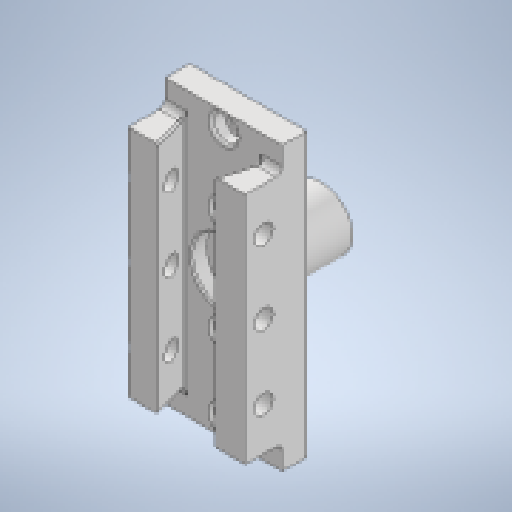
# Autodesk Inventor part: finger_adaptor
Saved by Autodesk Inventor 2024.3 (Build 283343010, 343A)
## iProperties
Created: 2025-06-26
Part Number: finger_adaptor
Material: 一般
Document SubType Name: Modeling
Designer: kshau
Density: 1 g/cm^3
Appearance: 滑らか - 黒
Author: kshau
Autodesk Inventor part; units mm, degrees
ref_plane "YZ Plane" through (0, 0, 0) normal (1, 0, 0) x (0, 1, 0)
ref_plane "XZ Plane" through (0, 0, 0) normal (0, 1, 0) x (-1, 0, 0)
ref_plane "XY Plane" through (0, 0, 0) normal (0, 0, 1) x (1, 0, 0)
sketch "スケッチ1" plane through (0, 0, 0) normal (0, 1, 0) x (-1, 0, 0)
  line L0 (0, 0) -> (19.05, 0)
  line L1 (19.05, 0) -> (19.05, 10)
  line L2 (19.05, 10) -> (0, 10)
  line L3 (0, 10) -> (0, 0)
  line L4 (19.05, 4) -> (0, 4)
  line L5 (14.265, 10) -> (15.873, 4)
  line L6 (9.525, 10) -> (9.525, 4)
  line L7 (0, 4) -> (19.05, 4)
  line L8 (4.785, 10) -> (3.177, 4)
  point P0 (3.177, 4)
  point P1 (4.785, 10)
  dimension "d0" = 19.05
  dimension "d1" = 10
  dimension "d2" = 4.785
  dimension "d3" = 4
  dimension "d4" = 3.177
  constraints: 18 end point, 5 point on line, 4 symmetric about line, 2 midpoint, 2 parallel, 2 perpendicular, 1 horizontal
  measures "d0" distance of L0.start L0.end
  measures "d1" distance of L0.end L1.end
  measures "d2" distance from line of L1 L5.start
  measures "d3" distance between parallel lines of L4 L0
  measures "d4" distance from line of L1 L5.end
extrude "押し出し1" add sketch "スケッチ1" along normal blind 46 contours L3 L4 L1 L0 | L3 L2 L8 L4 | L4 L5 L2 L1
sketch "スケッチ2" plane through (0, 0, 0) normal (0, 0, -1) x (-1, 0, 0)
  line L0 (15.873, 46) -> (3.177, 46) projected
  line L1 (9.525, 46) -> (9.525, 0)
  line L2 (15.873, 0) -> (3.177, 0) projected
  circle A0 centre (9.525, 23) radius 5
  point P0 (0, 0)
  dimension "d7" = 10
  constraints: 3 midpoint, 2 end point, 1 centre point
  measures "d7" diameter of A0
extrude "押し出し2" add sketch "スケッチ2" along normal blind 12.5
sketch "スケッチ3" plane through (-9.525, 23, -12.5) normal (0, 0, -1) x (-1, 0, 0)
  circle A0 centre (0, 0) radius 5 projected
  point P0 (-9.525, -23)
  constraints: 1 coincident
hole "穴1" at (-9.525, 23, -12.5) direction (0, 0, 1) diameter 3.1 end through all
sketch "スケッチ4" plane through (0, 0, 0) normal (0, 0, -1) x (-1, 0, 0)
  line L0 (15.873, 46) -> (3.177, 46) projected
  line L1 (9.525, 46) -> (9.525, 0)
  line L2 (15.873, 0) -> (3.177, 0) projected
  line L3 (0, 0) -> (0, 46) projected
  line L4 (0, 23) -> (19.05, 23)
  line L5 (19.05, 0) -> (19.05, 46) projected
  point P0 (9.525, 43.5)
  point P1 (9.525, 31.5)
  point P2 (9.525, 2.5)
  point P3 (9.525, 14.5)
  dimension "d17" = 2.5
  dimension "d18" = 12
  constraints: 4 end point, 4 midpoint, 2 point on line, 2 symmetric about line
  measures "d17" distance from line of L0 point (9.525, 43.5)
  measures "d18" distance of point (9.525, 43.5) point (9.525, 31.5)
hole "穴2" at (-9.525, 43.5, 0) at (-9.525, 31.5, 0) at (-9.525, 2.5, 0) at (-9.525, 14.5, 0) direction (0, 0, 1) diameter 2.1 end through all
sketch "スケッチ5" plane through (-19.05, 0, 0) normal (-1, 0, 0) x (0, 0, 1)
  line L0 (0, 46) -> (10, 46) projected
  line L1 (7, 46) -> (7, 0)
  line L2 (10, 0) -> (10, 46) projected
  line L3 (0, 0) -> (10, 0) projected
  line L4 (7, 23) -> (10, 23)
  point P0 (7, 11)
  point P1 (7, 35)
  dimension "d26" = 3
  dimension "d29" = 12
  constraints: 4 end point, 2 midpoint, 2 point on line, 1 coincident, 1 perpendicular, 1 symmetric about line, 1 vertical
  measures "d26" distance between parallel lines of L2 L1
  measures "d29" distance from line of point (7, 11) L4
hole "穴3" at (-19.05, 11, 7) at (-19.05, 23, 7) at (-19.05, 35, 7) direction (1, 0, 0) diameter 3.1 end through all countersink diameter 6.3 countersink angle 90
sketch "スケッチ6" plane through (-15.873, 0, 4) normal (0, 0, 1) x (1, 0, 0)
  circle A0 centre (6.348, 43.5) radius 1.05 projected
  circle A1 centre (6.348, 43.5) radius 2
  circle A2 centre (6.348, 31.5) radius 1.05 projected
  circle A3 centre (6.348, 31.5) radius 2
  circle A4 centre (6.348, 23) radius 1.55 projected
  circle A5 centre (6.348, 23) radius 3
  circle A6 centre (6.348, 14.5) radius 1.05 projected
  circle A7 centre (6.348, 14.5) radius 2
  circle A8 centre (6.348, 2.5) radius 1.05 projected
  circle A9 centre (6.348, 2.5) radius 2
  point P0 (15.873, 0)
  dimension "d37" = 4
  dimension "d38" = 4
  dimension "d39" = 6
  dimension "d40" = 4
  dimension "d41" = 4
  constraints: 5 centre point, 5 coincident
  measures "d37" diameter of A1
  measures "d38" diameter of A3
  measures "d39" diameter of A5
  measures "d40" diameter of A7
  measures "d41" diameter of A9
extrude "押し出し3" cut sketch "スケッチ6" against normal blind 2.1 contours A0 | A1 | A2 | A3 | A7 | A9
sketch "スケッチ7" plane through (0, 46, 0) normal (0, 1, 0) x (1, 0, 0)
  line L0 (-19.05, -10) -> (-14.265, -10) projected
  line L1 (-19.05, -10) -> (0, -10)
  line L2 (0, -10) -> (0, 0)
  line L3 (0, 0) -> (-19.05, 0)
  line L4 (-19.05, 0) -> (-19.05, -10)
  line L5 (-19.05, -4) -> (0, -4)
  line L6 (0, -10) -> (0, 0) projected
  point P0 (0, -4)
  dimension "d44" = 4
  constraints: 10 end point, 2 parallel, 2 perpendicular, 2 point on line, 1 horizontal
  measures "d44" distance between parallel lines of L3 L5
extrude "押し出し4" cut sketch "スケッチ7" against normal blind 3.95 contours L4 L5 L2 L1 L0
sketch "スケッチ8" plane through (0, 0, 0) normal (0, -1, 0) x (1, 0, 0)
  line L0 (0, 10) -> (0, 0) projected
  line L1 (0, 0) -> (-19.05, 0) projected
  line L2 (0, 10) -> (-19.05, 10)
  line L3 (-19.05, 10) -> (-19.05, 0)
  line L4 (-19.05, 0) -> (0, 0)
  line L5 (0, 0) -> (0, 10)
  line L6 (-19.05, 4) -> (-15.873, 4) projected
  line L7 (-19.05, 4) -> (0, 4)
  constraints: 10 end point, 2 parallel, 2 perpendicular, 1 horizontal, 1 point on line
extrude "押し出し5" cut sketch "スケッチ8" against normal blind 3.95 contours L0 L7 L6 L3 L2
fillet "フィレット1" radius 0.5 4 edges at (-11.525, 2.5, 4) (-11.525, 14.5, 4) (-11.525, 31.5, 4) (-11.525, 43.5, 4)
sketch "スケッチ9" plane through (-3.177, 42.05, 4) normal (0, 0, 1) x (1, 0, 0)
  circle A0 centre (-6.348, -19.05) radius 1.55 projected
  circle A1 centre (-6.348, -19.05) radius 5.3116
  line L0 (-6.348, -19.05) -> (-3.6922, -14.45)
  line L1 (-6.348, -19.05) -> (-6.348, -13.7384)
  line L2 (-6.348, -19.05) -> (-9.0038, -14.45)
  line L3 (-9.0038, -14.45) -> (-3.6922, -14.45)
  line L4 (-11.6596, -19.05) -> (-9.0038, -14.45)
  line L5 (-9.0038, -23.65) -> (-11.6596, -19.05)
  line L6 (-3.6922, -23.65) -> (-9.0038, -23.65)
  line L7 (-1.0364, -19.05) -> (-3.6922, -23.65)
  line L8 (-3.6922, -14.45) -> (-1.0364, -19.05)
  circle A2 centre (-6.348, -19.05) radius 4.6
  point P0 (3.177, -42.05)
  point P1 (-1.0364, -19.05)
  point P2 (-5.573, -17.7077)
  point P3 (-7.123, -17.7077)
  point P4 (-9.0038, -14.45)
  point P5 (-11.6596, -19.05)
  point P6 (-9.0038, -23.65)
  point P7 (-3.6922, -14.45)
  point P8 (-3.6922, -14.45)
  point P9 (-1.0364, -19.05)
  point P10 (-1.0364, -19.05)
  point P11 (-9.0038, -23.65)
  point P12 (-9.0038, -23.65)
  point P13 (-9.0038, -14.45)
  point P14 (-9.0038, -14.45)
  point P15 (-9.0038, -14.45)
  dimension "d51" = 30
  dimension "d54" = 360
  dimension "d64" = 9.2
  constraints: 18 end point, 2 centre point, 2 coincident, 2 point on circle, 1 horizontal, 1 symmetric about line, 1 vertical, 19 other
  measures "d51" angle of L1 L0
  measures "d64" diameter of A2
extrude "押し出し6" cut sketch "スケッチ9" against normal blind 2.5
sketch "スケッチ10" plane through (-9.525, 23, -12.5) normal (0, 0, -1) x (-1, 0, 0)
  circle A0 centre (0, 0) radius 2.4
  circle A1 centre (0, 0) radius 5
  point P0 (-9.525, -23)
  dimension "d58" = 4.8
  constraints: 2 centre point, 1 coincident
  measures "d58" diameter of A0
extrude "押し出し7" cut sketch "スケッチ10" against normal blind 0.5
fillet "フィレット2" radius 0.5 1 edges at (-7.125, 23, -12)
sketch "スケッチ11" plane through (-9.525, 23, 1.5) normal (0, 0, 1) x (1, 0, 0)
  circle A0 centre (0, 0) radius 1.55 projected
  circle A1 centre (0, 0) radius 3.1
  point P0 (9.525, -23)
  dimension "d65" = 6.2
  constraints: 1 centre point, 1 coincident
  measures "d65" diameter of A1
extrude "押し出し8" cut sketch "スケッチ11" against normal blind 2.5
fillet "フィレット3" radius 0.3 1 edges at (-12.625, 23, 1.5)
fillet "フィレット4" radius 0.3 1 edges at (-4.2134, 23, 4)
fillet "フィレット5" radius 0.3 2 edges at (-3.177, 23, 4) (-15.873, 23, 4)
fillet "フィレット6" radius 1 8 edges at (-17.4615, 42.05, 4) (-15.6775, 42.05, 4) (-3.3725, 42.05, 4) (-1.5885, 42.05, 4) (-17.4615, 3.95, 4) (-15.6775, 3.95, 4) (-3.3725, 3.95, 4) (-1.5885, 3.95, 4)
fillet "フィレット7" radius 0.3 12 edges at (-3.3567, 3.8941, 4.6704) (-3.3407, 3.3944, 4.1042) (-4.115, 3.95, 7.5) (-15.6933, 3.8941, 4.6704) (-15.7093, 3.3944, 4.1042) (-14.935, 3.95, 7.5) (-15.6933, 42.1059, 4.6704) (-15.7093, 42.6056, 4.1042) (-14.935, 42.05, 7.5) (-3.3567, 42.1059, 4.6704) (-3.3407, 42.6056, 4.1042) (-4.115, 42.05, 7.5)
fillet "フィレット8" radius 1.5 1 edges at (-4.525, 23, 0)
